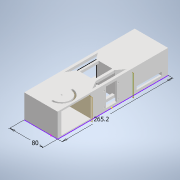
# Autodesk Inventor part: Part1
Saved by Autodesk Inventor 2022 (Build 260153000, 153)
## iProperties
Created: 2022-04-28
Part Number: Part1
Material: Generic
Document SubType Name: Modeling
Designer: Oana
Density: 1 g/cm^3
Appearance: Default
Author: Oana
Autodesk Inventor part; units mm, degrees
sketch "Sketch1" plane through (0, 0, 0) normal (0, 1, 0) x (-1, 0, 0)
  line L0 (49.8413, 129.2399) -> (-30.1587, 129.2399)
  line L1 (-30.1587, 129.2399) -> (-30.1587, -135.9601)
  line L2 (-30.1587, -135.9601) -> (49.8413, -135.9601)
  line L3 (49.8413, -135.9601) -> (49.8413, 129.2399)
  point P0 (0, 0)
  dimension "d0" = 265.2
  dimension "d1" = 80
  constraints: 8 end point, 2 parallel, 1 horizontal, 1 perpendicular
  measures "d0" distance of L0.end L1.end
  measures "d1" distance of L0.start L0.end
extrude "Extrusion1" add sketch "Sketch1" along normal blind 57
sketch "Sketch2" plane through (0, 0, 0) normal (0, -1, 0) x (1, 0, 0)
  line L0 (30.1587, 129.2399) -> (-49.8413, -135.9601) construction
  line L1 (30.1587, 129.2399) -> (30.1587, -135.9601) projected
  line L2 (-49.8413, 129.2399) -> (30.1587, 129.2399) projected
  line L3 (-49.8413, -135.9601) -> (-49.8413, 129.2399) projected
  line L4 (30.1587, -135.9601) -> (-49.8413, -135.9601) projected
  line L5 (-49.8413, 129.2399) -> (30.1587, -135.9601) construction
  line L6 (12.6587, 19.1399) -> (-32.3413, 19.1399)
  line L7 (-32.3413, 19.1399) -> (-32.3413, -25.8601)
  line L8 (-32.3413, -25.8601) -> (12.6587, -25.8601)
  line L9 (12.6587, -25.8601) -> (12.6587, 19.1399)
  line L10 (12.6587, 19.1399) -> (-32.3413, -25.8601) construction
  line L11 (-32.3413, 19.1399) -> (12.6587, -25.8601) construction
  point P0 (0, 0)
  point P1 (-9.8413, -3.3601)
  point P2 (-9.8413, -3.3601)
  dimension "d4" = 45
  dimension "d5" = 45
  constraints: 16 end point, 4 midpoint, 2 coincident, 2 parallel, 1 horizontal, 1 perpendicular
  measures "d4" distance of L6.start L6.end
  measures "d5" distance of L6.end L7.end
extrude "Extrusion2" cut sketch "Sketch2" against normal up to surface (57 mm away) contours L9 L8 L7 L6
sketch "Sketch6" plane through (0, 0, 0) normal (0, -1, 0) x (1, 0, 0)
  point P0 (0, 0)
sketch "Sketch7" plane through (0, 0, 0) normal (0, -1, 0) x (1, 0, 0)
  line L0 (12.4515, 19.3223) -> (12.4515, -25.5803)
  line L1 (12.4515, -25.5803) -> (30.1794, -49.7663)
  line L2 (30.1794, -49.7663) -> (30.1794, 50.0541)
  line L3 (30.1794, 50.0541) -> (12.4515, 19.3223)
  line L4 (-32.3413, 19.1399) -> (12.6587, 19.1399) projected
  line L5 (12.6587, 19.1399) -> (12.6587, -25.8601) projected
  line L6 (12.6587, -25.8601) -> (-32.3413, -25.8601) projected
  line L7 (-32.3413, -25.8601) -> (-32.3413, 19.1399) projected
  line L8 (30.1587, 129.2399) -> (30.1587, -135.9601) projected
  line L9 (-49.8413, 129.2399) -> (30.1587, 129.2399) projected
  line L10 (-49.8413, -135.9601) -> (-49.8413, 129.2399) projected
  line L11 (30.1587, -135.9601) -> (-49.8413, -135.9601) projected
  line L12 (-49.8413, 129.2399) -> (-49.8413, -135.9601)
  line L13 (-49.8413, -135.9601) -> (-49.8413, 129.2399) projected
  point P0 (0, 0)
  point P1 (12.6565, -25.8601)
  point P2 (30.1587, -49.7381)
  point P3 (30.1587, 50.0182)
  point P4 (12.4515, 19.1399)
  constraints: 10 end point, 1 collinear, 1 parallel, 1 vertical
extrude "Extrusion3" cut sketch "Sketch7" against normal up to surface (57 mm away) contours L3 L8 L1 L5 L4 L0
sketch "Sketch8" plane through (-32.3413, 0, 19.1399) normal (0, 0, -1) x (-1, 0, 0)
  line L0 (-44.7927, 0) -> (-38.7927, 0)
  line L1 (-38.7927, 0) -> (-38.7927, 6)
  line L2 (-38.7927, 6) -> (-44.7927, 6)
  line L3 (-44.7927, 6) -> (-44.7927, 0)
  line L4 (-44.7927, 51) -> (-38.7927, 51)
  line L5 (-38.7927, 51) -> (-38.7927, 57)
  line L6 (-38.7927, 57) -> (-44.7927, 57)
  line L7 (-44.7927, 57) -> (-44.7927, 51)
  line L8 (0, 0) -> (-44.7927, 0) projected
  point P0 (-32.3413, 0)
  dimension "d12" = 6
  dimension "d13" = 6
  constraints: 16 end point, 5 parallel, 2 equal length, 2 horizontal, 2 perpendicular, 2 point on line, 1 coincident
  measures "d12" distance of L0.end L1.end
  measures "d13" distance of L1.end L2.end
extrude "Extrusion4" add sketch "Sketch8" along normal up to surface (45 mm away)
sketch "Sketch9" plane through (-32.3413, 0, 19.1399) normal (1, 0, 0) x (0, 0, -1)
  line L0 (0, 57) -> (45, 57) projected
  line L1 (0, 0) -> (0, 57) projected
  line L2 (45, 0) -> (0, 0) projected
  line L3 (45, 0) -> (45, 57) projected
  line L4 (0, 0) -> (45, 0)
  line L5 (45, 0) -> (45, 57)
  line L6 (45, 57) -> (0, 57)
  line L7 (0, 57) -> (0, 0)
  point P0 (19.1399, 0)
  constraints: 8 end point, 2 parallel, 1 horizontal, 1 perpendicular
sketch "Sketch10" plane through (0, 0, 0) normal (0, -1, 0) x (1, 0, 0)
  line L0 (6.4515, -25.8601) -> (-32.3413, -25.8601) projected
  line L1 (-32.3413, -25.8601) -> (-32.3413, 19.1399) projected
  line L2 (-32.3413, 19.1399) -> (6.4515, 19.1399) projected
  line L3 (6.4515, 19.1399) -> (6.4515, -25.8601) projected
  line L4 (12.4515, -25.8601) -> (12.4515, 19.3223) projected
  line L5 (12.4515, 19.3223) -> (30.1587, 50.0182) projected
  line L6 (30.1587, 129.2399) -> (30.1587, 50.0182) projected
  line L7 (-49.8413, 129.2399) -> (30.1587, 129.2399) projected
  line L8 (-49.8413, -135.9601) -> (-49.8413, 129.2399) projected
  line L9 (30.1587, -135.9601) -> (-49.8413, -135.9601) projected
  line L10 (30.1587, -49.7381) -> (30.1587, -135.9601) projected
  line L11 (30.1587, -49.7381) -> (12.6565, -25.8601) projected
  line L12 (12.6565, -25.8601) -> (12.4515, -25.8601) projected
  line L13 (30.1587, 50.0182) -> (-49.8413, 50.0182) construction
  line L14 (30.1587, -49.7381) -> (-49.8413, -49.7381) construction
  line L15 (-32.3413, -25.8601) -> (-49.8413, -49.7381)
  line L16 (-49.8413, 50.0182) -> (-32.3413, 19.1399)
  line L17 (-49.8413, 50.0182) -> (-49.8413, -49.7381)
  point P0 (0, 0)
  constraints: 10 end point, 3 perpendicular, 2 point on line
extrude "Extrusion5" cut sketch "Sketch10" against normal up to surface (57 mm away) contours L15 L8 L16 L1
sketch "Sketch11" plane through (12.4515, 51, 19.1399) normal (0, 0, -1) x (-1, 0, 0)
  line L0 (44.7927, -51) -> (38.7927, -51)
  line L1 (38.7927, -51) -> (38.7927, -45)
  line L2 (38.7927, -45) -> (44.7927, -45)
  line L3 (44.7927, -45) -> (44.7927, -51)
  line L4 (44.7927, 6) -> (38.7927, 6)
  line L5 (38.7927, 6) -> (38.7927, 0)
  line L6 (38.7927, 0) -> (44.7927, 0)
  line L7 (44.7927, 0) -> (44.7927, 6)
  point P0 (12.4515, -51)
  dimension "d18" = 6
  dimension "d19" = 6
  dimension "d20" = 6
  dimension "d21" = 6
  constraints: 16 end point, 4 parallel, 2 horizontal, 2 perpendicular, 1 coincident
  measures "d18" distance of L0.end L1.end
  measures "d19" distance of L1.end L2.end
  measures "d20" distance of L4.end L5.end
  measures "d21" distance of L5.end L6.end
extrude "Extrusion6" add sketch "Sketch11" along normal up to surface (45 mm away)
ref_plane "Work Plane4" through (30.1587, 0, -49.7381) normal (0, 0, -1) x (0, -1, 0)
ref_plane "Work Plane5" through (30.1587, 0, 50.0182) normal (0, 0, 1) x (0, 1, 0)
sketch "Sketch14" plane through (30.1587, 0, -49.7381) normal (0, 0, -1) x (0, -1, 0)
  line L0 (-57, 17.5022) -> (-57, 0) projected
  line L1 (0, 17.5022) -> (-57, 17.5022) projected
  line L2 (0, 0) -> (0, 17.5022) projected
  line L3 (-57, 0) -> (0, 0) projected
  line L4 (-57, 0) -> (-51, 0)
  line L5 (-51, 0) -> (-51, 6)
  line L6 (-51, 6) -> (-57, 6)
  line L7 (-57, 6) -> (-57, 0)
  line L8 (-6, 0) -> (0, 0)
  line L9 (0, 0) -> (0, 6)
  line L10 (0, 6) -> (-6, 6)
  line L11 (-6, 6) -> (-6, 0)
  line L12 (0, 80) -> (-6, 80)
  line L13 (-6, 80) -> (-6, 74)
  line L14 (-6, 74) -> (0, 74)
  line L15 (0, 74) -> (0, 80)
  line L16 (-51, 80) -> (-57, 80)
  line L17 (-57, 80) -> (-57, 74)
  line L18 (-57, 74) -> (-51, 74)
  line L19 (-51, 74) -> (-51, 80)
  point P0 (0, 30.1587)
  dimension "d26" = 6
  dimension "d27" = 6
  dimension "d28" = 6
  dimension "d29" = 6
  constraints: 32 end point, 8 parallel, 8 perpendicular, 4 horizontal, 2 coincident
  measures "d26" distance of L4.end L5.end
  measures "d27" distance of L2.start L9.end
  measures "d28" distance of L12.end L13.end
  measures "d29" distance of L16.end L17.end
extrude "Extrusion7" add sketch "Sketch14" against normal up to surface (99.7563 mm away) contours L6 L5 L3 L0 | L2 L3 L11 L10 | L15 L14 L13 L12 | L19 L18 L17 L16
sketch "Sketch21" plane through (0, 0, 0) normal (0, -1, 0) x (1, 0, 0)
  arc A0 (-47.9413, -132.9601) -> (-44.9413, -135.9601) centre (-44.9413, -132.9601) ccw projected
  line L0 (-44.9413, -135.9601) -> (5.0587, -135.9601) projected
  arc A1 (5.0587, -135.9601) -> (8.0587, -132.9601) centre (5.0587, -132.9601) ccw projected
  line L1 (8.0587, -132.9601) -> (8.0587, -53.9601) projected
  arc A2 (8.0587, -53.9601) -> (5.0587, -50.9601) centre (5.0587, -53.9601) ccw projected
  line L2 (5.0587, -50.9601) -> (-44.9413, -50.9601) projected
  arc A3 (-44.9413, -50.9601) -> (-47.9413, -53.9601) centre (-44.9413, -53.9601) ccw projected
  line L3 (-47.9413, -53.9601) -> (-47.9413, -132.9601) projected
  spline S0 degree 3 poles (-15.1644, -62.5888) (-14.9628, -63.1953) (-14.6769, -64.3948) (-15.1993, -65.5952) (-15.7394, -65.8388) knots 0 0 0 0 0.539089 1 1 1 1 projected
  spline S1 degree 3 poles (-15.7394, -65.8388) (-14.4693, -66.5079) (-14.7995, -68.1116) (-15.2394, -69.1388) knots 0 0 0 0 1 1 1 1 projected
  spline S2 degree 3 poles (-15.2394, -69.1388) (-16.1604, -69.2836) (-17.1544, -68.892) (-17.7144, -68.1388) knots 0 0 0 0 1 1 1 1 projected
  spline S3 degree 3 poles (-17.7144, -68.1388) (-17.9663, -68.6471) (-18.6013, -68.8732) (-19.1394, -68.7888) knots 0 0 0 0 1 1 1 1 projected
  spline S4 degree 3 poles (-19.1394, -68.7888) (-19.3594, -69.0176) (-20.0467, -69.6983) (-21.1976, -69.5489) (-21.5644, -69.0067) knots 0 0 0 0 0.345385 1 1 1 1 projected
  spline S5 degree 3 poles (-21.5644, -69.0067) (-21.9665, -68.9706) (-23.0457, -68.9083) (-23.514, -67.8261) (-23.7411, -67.3609) knots 0 0 0 0 0.419509 1 1 1 1 projected
  spline S6 degree 3 poles (-23.7411, -67.3609) (-24.0812, -66.9137) (-24.6116, -66.2331) (-24.5516, -64.8465) (-23.8079, -64.3989) (-23.6675, -63.9025) knots 0 0 0 0 0.443124 0.609881 1 1 1 1 projected
  spline S7 degree 3 poles (-23.6675, -63.9025) (-23.3929, -62.9134) (-22.3359, -62.5853) (-21.4542, -62.4791) knots 0 0 0 0 1 1 1 1 projected
  spline S8 degree 3 poles (-21.4542, -62.4791) (-21.1982, -62.1521) (-20.2445, -61.9787) (-19.4136, -62.3867) (-19.1394, -62.8138) knots 0 0 0 0 0.450152 1 1 1 1 projected
  spline S9 degree 3 poles (-19.1394, -62.8138) (-18.555, -62.7473) (-17.9628, -63.0855) (-17.6144, -63.5388) knots 0 0 0 0 1 1 1 1 projected
  spline S10 degree 3 poles (-17.6144, -63.5388) (-17.3473, -63.1639) (-16.5978, -62.576) (-15.6276, -62.4003) (-15.1644, -62.5888) knots 0 0 0 0 0.487296 1 1 1 1 projected
  circle A4 centre (-2.8513, -113.7301) radius 0.8 projected
  circle A5 centre (-2.8513, -111.1901) radius 0.8 projected
  line L4 (0.4887, -111.9901) -> (-1.1113, -111.9901) projected
  line L5 (-1.1113, -111.9901) -> (-1.1113, -110.3901) projected
  line L6 (-1.1113, -110.3901) -> (0.4887, -110.3901) projected
  line L7 (0.4887, -110.3901) -> (0.4887, -111.9901) projected
  circle A6 centre (-0.3113, -113.7301) radius 0.8 projected
  line L8 (1.8687, -57.9101) -> (7.2487, -57.9101) projected
  line L9 (7.2487, -57.9101) -> (7.2487, -109.0101) projected
  line L10 (7.2487, -109.0101) -> (2.3859, -109.0101) projected
  line L11 (2.3859, -109.0101) -> (1.8687, -108.4929) projected
  line L12 (1.8687, -108.4929) -> (1.8687, -57.9101) projected
  circle A7 centre (-44.4413, -112.4601) radius 3 projected
  circle A8 centre (-44.4413, -54.4601) radius 3 projected
  circle A9 centre (4.5587, -54.4601) radius 3 projected
  circle A10 centre (4.5587, -112.4601) radius 3 projected
  line L13 (24.1587, -41.5524) -> (12.6565, -25.8601) projected
  line L14 (12.6565, -25.8601) -> (12.4515, -25.8601) projected
  line L15 (12.4515, -25.8601) -> (12.4515, 19.3223) projected
  line L16 (12.4515, 19.3223) -> (24.1587, 39.6171) projected
  line L17 (24.1587, -41.5524) -> (24.1587, 39.6171) projected
  line L18 (-43.8413, 39.4314) -> (-32.3413, 19.1399) projected
  line L19 (-32.3413, 19.1399) -> (-32.3413, -25.8601) projected
  line L20 (-32.3413, -25.8601) -> (-43.8413, -41.5513) projected
  line L21 (-43.8413, -41.5513) -> (-43.8413, 39.4314) projected
  line L22 (-26.3413, 19.1399) -> (-26.3413, -25.8601) projected
  line L23 (-26.3413, 19.1399) -> (6.4515, 19.1399) projected
  line L24 (6.4515, 19.1399) -> (6.4515, -25.8601) projected
  line L25 (6.4515, -25.8601) -> (-26.3413, -25.8601) projected
  line L26 (30.1587, 129.2399) -> (30.1587, -135.9601) projected
  line L27 (-49.8413, 129.2399) -> (30.1587, 129.2399) projected
  line L28 (-49.8413, -135.9601) -> (-49.8413, 129.2399) projected
  line L29 (30.1587, -135.9601) -> (-49.8413, -135.9601) projected
  line L30 (-49.8413, -45.9601) -> (20.1587, -45.9601)
  line L31 (20.1587, -45.9601) -> (20.1587, -135.9601)
  line L32 (20.1587, -135.9601) -> (-49.8413, -135.9601)
  line L33 (-49.8413, -135.9601) -> (-49.8413, -45.9601)
  point P0 (0, 0)
  dimension "d45" = 90
  dimension "d56" = 70
  constraints: 8 end point, 2 parallel, 2 point on line, 1 horizontal, 1 perpendicular
  measures "d45" distance of L30.end L31.end
  measures "d56" distance of L30.start L30.end
extrude "Extrusion12" cut sketch "Sketch21" against normal blind 25 contours L3 A3 L2 A2 L1 A1 L0 A0 | A0 L29 L28 L30 L31 A1 L1 A2 L2 A3 L3 | S0 S1 S2 S3 S4 S5 S6 S7 S8 S9 S10 | A4 | A5 | L4 L5 L6 L7 | A6 | L8 L9 L10 L11 L12 | A7 | A8 | A9 | A10
sketch "Sketch24" plane through (0, 0, 0) normal (0, -1, 0) x (1, 0, 0)
  line L0 (20.1587, -45.9601) -> (20.1587, -135.9601) projected
  line L1 (30.1587, -135.9601) -> (20.1587, -135.9601) projected
  line L2 (30.1587, 129.2399) -> (30.1587, -135.9601) projected
  line L3 (-49.8413, 129.2399) -> (30.1587, 129.2399) projected
  line L4 (-49.8413, -45.9601) -> (-49.8413, 129.2399) projected
  line L5 (-49.8413, -45.9601) -> (20.1587, -45.9601) projected
  line L6 (24.1587, -41.5524) -> (12.6565, -25.8601) projected
  line L7 (12.6565, -25.8601) -> (12.4515, -25.8601) projected
  line L8 (12.4515, -25.8601) -> (12.4515, 19.3223) projected
  line L9 (12.4515, 19.3223) -> (24.1587, 39.6171) projected
  line L10 (24.1587, -41.5524) -> (24.1587, 39.6171) projected
  line L11 (-43.8413, 39.4314) -> (-32.3413, 19.1399) projected
  line L12 (-32.3413, 19.1399) -> (-32.3413, -25.8601) projected
  line L13 (-32.3413, -25.8601) -> (-43.8413, -41.5513) projected
  line L14 (-43.8413, -41.5513) -> (-43.8413, 39.4314) projected
  line L15 (-26.3413, 19.1399) -> (-26.3413, -25.8601) projected
  line L16 (-26.3413, 19.1399) -> (6.4515, 19.1399) projected
  line L17 (6.4515, 19.1399) -> (6.4515, -25.8601) projected
  line L18 (6.4515, -25.8601) -> (-26.3413, -25.8601) projected
  line L19 (20.1587, -45.9601) -> (26.1587, -45.9601)
  line L20 (26.1587, -45.9601) -> (26.1587, -135.9601)
  line L21 (26.1587, -135.9601) -> (20.1587, -135.9601)
  line L22 (20.1587, -135.9601) -> (20.1587, -45.9601)
  point P0 (0, 0)
  dimension "d46" = 6
  constraints: 8 end point, 2 parallel, 1 horizontal, 1 perpendicular, 1 point on line
  measures "d46" distance between parallel lines of L20 L0
extrude "Extrusion13" cut sketch "Sketch24" against normal blind 7 contours L19 L20 L1 L0
ref_plane "Work Plane6" through (6.4515, 8.5, -23.3601) normal (1, 0, 0) x (0, 1, 0)
sketch "Sketch27" plane through (6.4515, 0, -25.8601) normal (-1, 0, 0) x (0, 0, 1)
  circle A0 centre (38.4706, 10.5294) radius 1 projected
  circle A1 centre (4.5294, 10.5294) radius 1 projected
  circle A2 centre (4.5294, 44.4706) radius 1 projected
  circle A3 centre (38.4706, 44.4706) radius 1 projected
  arc A4 (37.2331, 41.4654) -> (35.4654, 43.2331) centre (36.3492, 42.3492) ccw projected
  arc A5 (35.1118, 42.8796) -> (36.8796, 41.1118) centre (35.9957, 41.9957) ccw projected
  line L0 (37.2331, 41.4654) -> (36.8796, 41.1118) projected
  line L1 (35.1118, 42.8796) -> (35.4654, 43.2331) projected
  arc A6 (6.1204, 41.1118) -> (7.8882, 42.8796) centre (7.0043, 41.9957) ccw projected
  line L2 (6.1204, 41.1118) -> (5.7669, 41.4654) projected
  arc A7 (7.5346, 43.2331) -> (5.7669, 41.4654) centre (6.6508, 42.3492) ccw projected
  line L3 (7.5346, 43.2331) -> (7.8882, 42.8796) projected
  arc A8 (5.7669, 13.5346) -> (7.5346, 11.7669) centre (6.6508, 12.6508) ccw projected
  arc A9 (7.8882, 12.1204) -> (6.1204, 13.8882) centre (7.0043, 13.0043) ccw projected
  line L4 (5.7669, 13.5346) -> (6.1204, 13.8882) projected
  line L5 (7.8882, 12.1204) -> (7.5346, 11.7669) projected
  arc A10 (35.4654, 11.7669) -> (37.2331, 13.5346) centre (36.3492, 12.6508) ccw projected
  arc A11 (36.8796, 13.8882) -> (35.1118, 12.1204) centre (35.9957, 13.0043) ccw projected
  line L6 (35.4654, 11.7669) -> (35.1118, 12.1204) projected
  line L7 (36.8796, 13.8882) -> (37.2331, 13.5346) projected
  point P0 (25.8601, 0)
  constraints: 1 other
extrude "Extrusion16" cut sketch "Sketch27" against normal up to surface (6 mm away)
sketch "Sketch28" plane through (30.1587, 0, 129.2399) normal (1, 0, 0) x (0, 0, -1)
  point P0 (129.2399, 0)
sketch "Sketch29" plane through (0, 25, 0) normal (0, -1, 0) x (1, 0, 0)
  line L0 (-49.8413, -49.7381) -> (-47.0724, -45.9601) projected
  line L1 (-49.8413, -135.9601) -> (-49.8413, -49.7381) projected
  line L2 (20.1587, -135.9601) -> (-49.8413, -135.9601) projected
  line L3 (20.1587, -45.9601) -> (20.1587, -135.9601) projected
  line L4 (-47.0724, -45.9601) -> (20.1587, -45.9601) projected
  line L5 (-49.8413, -135.9601) -> (-44.8413, -135.9601)
  line L6 (-44.8413, -135.9601) -> (-44.8413, -115.9601)
  line L7 (-49.8413, -120.9601) -> (-49.8413, -135.9601)
  line L8 (-49.8413, -49.7381) -> (-44.8413, -49.7381) construction
  line L9 (-44.8413, -49.7381) -> (-44.8413, -54.7381)
  line L10 (-49.8413, -54.7381) -> (-49.8413, -49.7381)
  line L11 (-49.8413, -49.7381) -> (-47.0724, -45.9601)
  line L12 (-44.8413, -45.9601) -> (-44.8413, -49.7381)
  line L13 (-44.8413, -115.9601) -> (-49.8413, -115.9601)
  line L14 (-44.8413, -54.7381) -> (-49.8413, -54.7381)
  line L15 (-37.0388, -135.9601) -> (-37.0388, -115.9601)
  line L16 (-37.0388, -115.9601) -> (-44.8413, -115.9601)
  line L17 (-44.8413, -135.9601) -> (-37.0388, -135.9601)
  point P0 (0, 0)
  dimension "d57" = 20
  dimension "d164" = 5
  dimension "d165" = 5
  dimension "d168" = 20
  constraints: 26 end point, 4 parallel, 4 perpendicular, 4 point on line, 3 horizontal, 2 vertical, 1 collinear
  measures "d57" distance of L5.end L6.end
  measures "d164" distance of L6.end L13.end
  measures "d165" distance of L8.end L9.end
  measures "d168" distance of L15.start L15.end
ref_plane "Work Plane7" through (-49.8413, 0, -135.9601) normal (0, -1, 0) x (1, 0, 0)
ref_plane "Work Plane8" through (-49.8413, 3, -135.9601) normal (0, 1, 0) x (0, 0, 1)
ref_plane "Work Plane9" through (-49.8413, 3, -135.9601) normal (0, 1, 0) x (0, 0, 1)
extrude "Extrusion19" add sketch "Sketch29" along normal up to surface (22 mm away) contours L0 L4 L12 L9 L14 L1 | L13 L6 L2 L1 | L16 L15 L2 L6
sketch "Sketch34" plane through (0, 25, 0) normal (0, -1, 0) x (1, 0, 0)
  circle A0 centre (-32.3413, -111.4601) radius 1.35 projected
  circle A1 centre (-32.3413, -53.4601) radius 1.35 projected
  circle A2 centre (16.6587, -53.4601) radius 1.35 projected
  circle A3 centre (16.6587, -111.4601) radius 1.35 projected
  point P0 (0, 0)
extrude "Extrusion21" cut sketch "Sketch34" against normal blind 12
sketch "Sketch38" plane through (30.1587, 0, 129.2399) normal (1, 0, 0) x (0, 0, -1)
  line L0 (69.2217, 3) -> (19.2217, 3)
  line L1 (19.2217, 3) -> (19.2217, 53)
  line L2 (19.2217, 53) -> (69.2217, 53)
  line L3 (69.2217, 53) -> (69.2217, 3)
  line L4 (0, 57) -> (265.2, 57) projected
  line L5 (0, 0) -> (0, 57) projected
  line L6 (0, 0) -> (265.2, 0) projected
  line L7 (265.2, 0) -> (265.2, 57) projected
  line L8 (178.978, 51) -> (79.2217, 51) projected
  line L9 (178.978, 51) -> (178.978, 6) projected
  line L10 (178.978, 6) -> (79.2217, 6) projected
  line L11 (79.2217, 6) -> (79.2217, 51) projected
  line L12 (64.2734, 53) -> (64.2734, 57)
  line L13 (79.2217, 20.8757) -> (69.2217, 20.8757)
  point P0 (129.2399, 0)
  dimension "d75" = 50
  dimension "d76" = 4
  dimension "d77" = 3
  dimension "d78" = 10
  constraints: 12 end point, 4 perpendicular, 4 point on line, 2 parallel, 1 horizontal
  measures "d75" distance of L1.end L2.end
  measures "d76" distance of L12.start L12.end
  measures "d77" distance between parallel lines of L6 L0
  measures "d78" distance of L13.start L13.end
extrude "Extrusion23" cut sketch "Sketch38" against normal up to surface (80 mm away) contours L0 L1 L2 L3
sketch "Sketch42" plane through (30.1587, 0, 129.2399) normal (1, 0, 0) x (0, 0, -1)
  line L0 (19.2217, 3) -> (19.2217, 53) projected
  line L1 (19.2217, 53) -> (69.2217, 53) projected
  line L2 (69.2217, 53) -> (69.2217, 3) projected
  line L3 (69.2217, 3) -> (19.2217, 3) projected
  line L4 (0, 57) -> (265.2, 57) projected
  line L5 (0, 0) -> (0, 57) projected
  line L6 (0, 0) -> (265.2, 0) projected
  line L7 (265.2, 0) -> (265.2, 57) projected
  line L8 (178.978, 51) -> (79.2217, 51) projected
  line L9 (178.978, 51) -> (178.978, 6) projected
  line L10 (178.978, 6) -> (79.2217, 6) projected
  line L11 (79.2217, 6) -> (79.2217, 51) projected
  line L12 (178.978, 0) -> (142.103, 0)
  line L13 (142.103, 0) -> (142.103, 57)
  line L14 (142.103, 57) -> (178.978, 57)
  line L15 (178.978, 57) -> (178.978, 0)
  line L16 (178.978, 26.2177) -> (178.978, 57)
  line L17 (116.0967, 0) -> (79.2217, 0)
  line L18 (79.2217, 0) -> (79.2217, 57)
  line L19 (79.2217, 57) -> (116.0967, 57)
  line L20 (116.0967, 57) -> (116.0967, 0)
  line L21 (79.2217, 28.5) -> (79.2217, 57)
  point P0 (129.2399, 0)
  point P1 (178.978, 6)
  dimension "d87" = 36.875
  constraints: 20 end point, 9 point on line, 4 parallel, 4 perpendicular, 2 horizontal, 1 collinear, 1 midpoint
  measures "d87" distance of L12.start L12.end
extrude "Extrusion26" add sketch "Sketch42" against normal blind 3 contours L4 L20 L8 L18 | L8 L20 L10 L11 | L18 L10 L20 L6 | L4 L15 L8 L13 | L8 L9 L10 L13 | L13 L10 L15 L6
sketch "Sketch43" plane through (30.1587, 0, 129.2399) normal (1, 0, 0) x (0, 0, -1)
  line L0 (142.103, 9.5) -> (146.074, 9.5)
  line L1 (0, 0) -> (265.2, 0) projected
  line L2 (142.103, 6) -> (142.103, 9.5)
  circle A0 centre (146.074, 9.5) radius 1.5
  point P0 (129.2399, 0)
  dimension "d90" = 3.971
  dimension "d91" = 3.5
  dimension "d92" = 3
  constraints: 4 end point, 2 coincident, 1 centre point, 1 horizontal, 1 parallel, 1 vertical
  measures "d90" distance of L0.start L0.end
  measures "d91" distance of L2.start L0.start
  measures "d92" diameter of A0
extrude "Extrusion27" cut sketch "Sketch43" against normal up to surface (3 mm away)
sketch "Sketch44" plane through (27.1587, 0, 129.2399) normal (-1, 0, 0) x (0, 0, 1)
  circle A0 centre (-112.1329, 9.5) radius 1 projected
  circle A1 centre (-112.1329, 43.4411) radius 1 projected
  point P0 (-129.2399, 0)
extrude "Extrusion28" cut sketch "Sketch44" against normal up to surface (3 mm away)
sketch "Sketch45" plane through (27.1587, 0, 129.2399) normal (-1, 0, 0) x (0, 0, 1)
  circle A0 centre (-146.074, 43.4411) radius 1 projected
  point P0 (-129.2399, 0)
extrude "Extrusion29" cut sketch "Sketch45" against normal up to surface (3 mm away)
sketch "Sketch54" plane through (30.1587, 0, 129.2399) normal (1, 0, 0) x (0, 0, -1)
  line L0 (249.9086, 6.9208) -> (189.9086, 6.9208)
  line L1 (189.9086, 6.9208) -> (189.9086, 14.9208)
  line L2 (189.9086, 14.9208) -> (249.9086, 14.9208)
  line L3 (249.9086, 14.9208) -> (249.9086, 6.9208)
  point P0 (129.2399, 0)
  dimension "d128" = 8
  dimension "d131" = 60
  constraints: 8 end point, 2 parallel, 1 horizontal, 1 perpendicular
  measures "d128" distance between parallel lines of L2 L0
  measures "d131" distance of L1.end L2.end
extrude "Extrusion37" cut sketch "Sketch54" against normal blind 10
sketch "Sketch55" plane through (30.1587, 0, 129.2399) normal (1, 0, 0) x (0, 0, -1)
  circle A0 centre (112.1329, 43.4411) radius 1 projected
  circle A1 centre (112.1329, 9.5) radius 1 projected
  circle A2 centre (146.074, 9.5) radius 1.5 projected
  circle A3 centre (146.074, 43.4411) radius 1 projected
  circle A4 centre (112.1329, 43.4411) radius 1.5
  circle A5 centre (112.1329, 9.5) radius 1.5
  circle A6 centre (146.074, 9.5) radius 1.5
  circle A7 centre (146.074, 43.4411) radius 1.5
  point P0 (129.2399, 0)
  dimension "d132" = 3
  dimension "d133" = 3
  dimension "d134" = 3
  dimension "d135" = 3
  constraints: 4 centre point, 4 coincident
  measures "d132" diameter of A4
  measures "d133" diameter of A5
  measures "d134" diameter of A6
  measures "d135" diameter of A7
extrude "Extrusion38" cut sketch "Sketch55" against normal up to surface (3 mm away) contours A0 | A1 | A2 | A3 | A4 | A5 | A7
sketch "Sketch56" plane through (30.1587, 0, 129.2399) normal (1, 0, 0) x (0, 0, -1)
  point P0 (129.2399, 0)
sketch "Sketch58" plane through (0, 0, 0) normal (0, -1, 0) x (1, 0, 0)
  line L0 (-15.7732, 129.2399) -> (-15.7732, 49.7366)
  line L1 (-49.8413, 129.2399) -> (30.1587, 129.2399) projected
  point P0 (0, 0)
  point P1 (15.1587, 129.2399)
  constraints: 2 end point, 1 point on line, 1 vertical
sketch "Sketch61" plane through (0, 57, 0) normal (0, 1, 0) x (1, 0, 0)
  line L0 (-43.8413, 41.5513) -> (-43.8413, -39.4314) projected
  line L1 (-43.8413, 41.5513) -> (-32.3413, 25.8601) projected
  line L2 (-32.3413, -19.1399) -> (-32.3413, 25.8601) projected
  line L3 (-32.3413, -19.1399) -> (-43.8413, -39.4314) projected
  line L4 (-26.3413, 25.8601) -> (6.4515, 25.8601) projected
  line L5 (6.4515, -19.1399) -> (6.4515, 25.8601) projected
  line L6 (6.4515, -19.1399) -> (-26.3413, -19.1399) projected
  line L7 (-26.3413, -19.1399) -> (-26.3413, 25.8601) projected
  line L8 (30.1587, -129.2399) -> (30.1587, 135.9601) projected
  line L9 (30.1587, 135.9601) -> (-49.8413, 135.9601) projected
  line L10 (-49.8413, 135.9601) -> (-49.8413, -129.2399) projected
  line L11 (-49.8413, -129.2399) -> (30.1587, -129.2399) projected
  line L12 (24.1587, -39.6171) -> (12.4515, -19.3223) projected
  line L13 (12.4515, -19.3223) -> (12.4515, 25.8601) projected
  line L14 (12.4515, 25.8601) -> (12.6565, 25.8601) projected
  line L15 (12.6565, 25.8601) -> (24.1587, 41.5524) projected
  line L16 (24.1587, 41.5524) -> (24.1587, -39.6171) projected
  line L17 (0.1587, -50.0182) -> (0.1587, -68.0309)
  line L18 (46.1587, -50.0182) -> (-65.8413, -50.0182) projected
  arc A0 (0.1587, -64.0309) -> (0.1587, -115.0309) centre (0.1587, -89.5309) ccw construction
  arc A1 (0.1587, -115.0309) -> (0.1587, -64.0309) centre (0.1587, -89.5309) ccw
  line L19 (0.1587, -115.0309) -> (0.1587, -129.2399)
  arc A2 (0.1587, -111.0309) -> (0.1587, -68.0309) centre (0.1587, -89.5309) ccw
  line L20 (0.1587, -68.0309) -> (0.1587, -115.0309)
  arc A3 (0.1587, -68.0309) -> (0.1587, -111.0309) centre (0.1587, -89.5309) ccw construction
  line L21 (0.1587, -68.0309) -> (0.1587, -64.0309)
  line L22 (0.1587, -115.0309) -> (0.1587, -111.0309)
  circle A4 centre (0.1587, -89.5309) radius 1.5
  point P0 (0, 0)
  dimension "d148" = 30
  dimension "d149" = 51
  dimension "d150" = 43
  dimension "d153" = 3
  dimension "d154" = 25.5
  constraints: 10 end point, 10 point on circle, 5 centre point, 4 point on line, 3 coincident, 3 perpendicular, 2 vertical
  measures "d148" distance between parallel lines of L17 L8
  measures "d149" distance of L19.start L21.end
  measures "d150" diameter of A2
  measures "d153" diameter of A4
  measures "d154" distance of A2.centre L21.end
extrude "Extrusion41" cut sketch "Sketch61" against normal up to surface (4 mm away) contours L20 A2 L17 A1 | A4 L20 | L20 A4
sketch "Sketch62" plane through (30.1587, 0, 129.2399) normal (1, 0, 0) x (0, 0, -1)
  circle A0 centre (112.1329, 43.4411) radius 1.5 projected
  circle A1 centre (146.074, 43.4411) radius 1.5 projected
  circle A2 centre (112.1329, 9.5) radius 1.5 projected
  line L0 (189.9086, 6.9208) -> (189.9086, 14.9208) projected
  line L1 (189.9086, 14.9208) -> (249.9086, 14.9208) projected
  line L2 (249.9086, 14.9208) -> (249.9086, 6.9208) projected
  line L3 (249.9086, 6.9208) -> (189.9086, 6.9208) projected
  circle A3 centre (146.074, 9.5) radius 1.5 projected
  line L4 (0, 0) -> (265.2, 0) projected
  line L5 (265.2, 0) -> (265.2, 57) projected
  line L6 (0, 57) -> (265.2, 57) projected
  line L7 (0, 0) -> (0, 57) projected
  line L8 (19.2217, 3) -> (19.2217, 53) projected
  line L9 (19.2217, 53) -> (69.2217, 53) projected
  line L10 (69.2217, 53) -> (69.2217, 3) projected
  line L11 (69.2217, 3) -> (19.2217, 3) projected
  line L12 (116.0967, 6) -> (116.0967, 51) projected
  line L13 (142.103, 51) -> (116.0967, 51) projected
  line L14 (142.103, 51) -> (142.103, 6) projected
  line L15 (142.103, 6) -> (116.0967, 6) projected
  line L16 (19.2217, 53) -> (9.2217, 53)
  line L17 (9.2217, 53) -> (9.2217, 3)
  line L18 (9.2217, 3) -> (19.2217, 3)
  line L19 (19.2217, 3) -> (19.2217, 53)
  point P0 (129.2399, 0)
  dimension "d155" = 10
  constraints: 8 end point, 2 parallel, 1 horizontal, 1 perpendicular
  measures "d155" distance of L17.end L18.end
extrude "Extrusion42" cut sketch "Sketch62" against normal up to surface (80 mm away) contours L18 L17 L16 L8
sketch "Sketch63" plane through (30.1587, 0, 50.0182) normal (0, 0, 1) x (0, 1, 0)
  point P0 (0, 30.1587)
sketch "Sketch64" plane through (30.1587, 0, 129.2399) normal (1, 0, 0) x (0, 0, -1)
  line L0 (116.0967, 6) -> (116.0967, 51) projected
  line L1 (142.103, 51) -> (116.0967, 51) projected
  line L2 (142.103, 51) -> (142.103, 6) projected
  line L3 (142.103, 6) -> (116.0967, 6) projected
  line L4 (69.2217, 3) -> (9.2217, 3) projected
  line L5 (9.2217, 3) -> (9.2217, 53) projected
  line L6 (9.2217, 53) -> (69.2217, 53) projected
  line L7 (69.2217, 53) -> (69.2217, 3) projected
  line L8 (0, 0) -> (265.2, 0) projected
  line L9 (265.2, 0) -> (265.2, 57) projected
  line L10 (0, 57) -> (265.2, 57) projected
  line L11 (0, 0) -> (0, 57) projected
  circle A0 centre (146.074, 9.5) radius 1.5 projected
  line L12 (189.9086, 6.9208) -> (189.9086, 14.9208) projected
  line L13 (189.9086, 14.9208) -> (249.9086, 14.9208) projected
  line L14 (249.9086, 14.9208) -> (249.9086, 6.9208) projected
  line L15 (249.9086, 6.9208) -> (189.9086, 6.9208) projected
  circle A1 centre (112.1329, 9.5) radius 1.5 projected
  circle A2 centre (146.074, 43.4411) radius 1.5 projected
  circle A3 centre (112.1329, 43.4411) radius 1.5 projected
  line L16 (69.2217, 53) -> (79.3445, 53)
  line L17 (79.3445, 53) -> (79.3445, 3)
  line L18 (79.3445, 3) -> (69.2217, 3)
  line L19 (69.2217, 3) -> (69.2217, 53)
  point P0 (129.2399, 0)
  constraints: 8 end point, 2 parallel, 1 horizontal, 1 perpendicular
extrude "Extrusion43" cut sketch "Sketch64" against normal up to surface (80 mm away) contours L7 L16 L17 L18
sketch "Sketch65" plane through (-49.8413, 0, 129.2399) normal (-1, 0, 0) x (0, 0, 1)
  circle A0 centre (-252.7, 22.2932) radius 2.5
  line L0 (-265.2, 57) -> (0, 57) projected
  line L1 (-265.2, 0) -> (0, 0) projected
  line L2 (-265.2, 3) -> (-265.2, 57) projected
  line L3 (-252.7, 22.2932) -> (-265.2, 22.2932)
  line L4 (-265.2, 22.2932) -> (-265.2, 28.2932)
  line L5 (-265.2, 28.2932) -> (-265.2, 28.2932)
  line L6 (-265.2, 28.2932) -> (-265.2, 34.2932)
  line L7 (-265.2, 34.2932) -> (-252.7, 34.2932)
  circle A1 centre (-252.7, 34.2932) radius 2.5
  point P0 (-129.2399, 0)
  dimension "d161" = 5
  dimension "d181" = 12.5
  dimension "d182" = 6
  dimension "d183" = 6
  dimension "d184" = 5
  constraints: 10 end point, 4 perpendicular, 4 point on line, 2 centre point, 1 coincident, 1 horizontal, 1 parallel, 1 vertical, 1 other
  measures "d161" diameter of A0
  measures "d181" distance of L3.start L3.end
  measures "d182" distance of L4.start L4.end
  measures "d183" distance of L4.end L6.end
  measures "d184" diameter of A1
extrude "Extrusion44" cut sketch "Sketch65" against normal blind 12
sketch "Sketch66" plane through (-49.8413, 0, 129.2399) normal (-1, 0, 0) x (0, 0, 1)
  circle A0 centre (-252.7, 22.2932) radius 2.5 projected
  line L0 (-79.3445, 3) -> (-79.3445, 6) projected
  line L1 (-175.2, 6) -> (-79.3445, 6) projected
  line L2 (-175.2, 6) -> (-175.2, 0) projected
  line L3 (-175.2, 0) -> (0, 0) projected
  line L4 (0, 0) -> (0, 57) projected
  line L5 (-265.2, 57) -> (0, 57) projected
  line L6 (-265.2, 3) -> (-265.2, 57) projected
  line L7 (-245.2, 3) -> (-265.2, 3) projected
  line L8 (-245.2, 25) -> (-245.2, 3) projected
  line L9 (-245.2, 25) -> (-183.978, 25) projected
  line L10 (-183.978, 25) -> (-183.978, 3) projected
  line L11 (-178.978, 3) -> (-183.978, 3) projected
  line L12 (-178.978, 3) -> (-178.978, 51) projected
  line L13 (-178.978, 51) -> (-79.3445, 51) projected
  line L14 (-79.3445, 51) -> (-79.3445, 53) projected
  line L15 (-79.3445, 53) -> (-9.2217, 53) projected
  line L16 (-9.2217, 53) -> (-9.2217, 3) projected
  line L17 (-9.2217, 3) -> (-79.3445, 3) projected
  line L18 (-9.2217, 29.5326) -> (-17.2217, 29.5326) construction
  line L19 (-17.2217, 29.5326) -> (-17.2217, 13.5326)
  line L20 (-17.2217, 13.5326) -> (-9.2217, 13.5326)
  line L21 (-9.2217, 13.5326) -> (-9.2217, 29.5326)
  line L22 (-9.2217, 29.5326) -> (-17.2217, 29.5326)
  line L23 (-17.2217, 29.5326) -> (-17.2217, 45.5326)
  line L24 (-17.2217, 45.5326) -> (-9.2217, 45.5326)
  line L25 (-9.2217, 45.5326) -> (-9.2217, 29.5326)
  point P0 (-129.2399, 0)
  point P1 (-9.2217, 13.5326)
  point P2 (-9.2217, 45.5326)
  dimension "d169" = 8
  dimension "d170" = 16
  constraints: 16 end point, 4 parallel, 2 horizontal, 2 perpendicular, 2 point on line, 1 collinear
  measures "d169" distance of L19.end L20.end
  measures "d170" distance of L18.end L19.end
extrude "Extrusion45" add sketch "Sketch66" against normal blind 30 contours L20 L19 L22 L16 | L22 L23 L24 L16
sketch "Sketch67" plane through (-49.8413, 0, 129.2399) normal (-1, 0, 0) x (0, 0, 1)
  circle A0 centre (-252.7, 22.2932) radius 2.5 projected
  line L0 (-79.3445, 3) -> (-79.3445, 6) projected
  line L1 (-175.2, 6) -> (-79.3445, 6) projected
  line L2 (-175.2, 6) -> (-175.2, 0) projected
  line L3 (-175.2, 0) -> (0, 0) projected
  line L4 (0, 0) -> (0, 57) projected
  line L5 (-265.2, 57) -> (0, 57) projected
  line L6 (-265.2, 3) -> (-265.2, 57) projected
  line L7 (-245.2, 3) -> (-265.2, 3) projected
  line L8 (-245.2, 25) -> (-245.2, 3) projected
  line L9 (-245.2, 25) -> (-183.978, 25) projected
  line L10 (-183.978, 25) -> (-183.978, 3) projected
  line L11 (-178.978, 3) -> (-183.978, 3) projected
  line L12 (-178.978, 3) -> (-178.978, 51) projected
  line L13 (-178.978, 51) -> (-79.3445, 51) projected
  line L14 (-79.3445, 51) -> (-79.3445, 53) projected
  line L15 (-79.3445, 53) -> (-9.2217, 53) projected
  line L16 (-9.2217, 53) -> (-9.2217, 45.5326) projected
  line L17 (-9.2217, 45.5326) -> (-17.2217, 45.5326) projected
  line L18 (-17.2217, 45.5326) -> (-17.2217, 13.5326) projected
  line L19 (-17.2217, 13.5326) -> (-9.2217, 13.5326) projected
  line L20 (-9.2217, 13.5326) -> (-9.2217, 3) projected
  line L21 (-9.2217, 3) -> (-79.3445, 3) projected
  line L22 (0, 30) -> (-12.5, 30)
  line L23 (-12.5, 30) -> (-12.5, 36)
  line L24 (-12.5, 36) -> (-12.5, 30)
  line L25 (-12.5, 30) -> (-12.5, 24)
  circle A1 centre (-12.5, 24) radius 2.5
  circle A2 centre (-12.5, 36) radius 2.5
  point P0 (-129.2399, 0)
  point P1 (-17.2217, 30)
  dimension "d173" = 12.5
  dimension "d175" = 6
  dimension "d176" = 6
  dimension "d177" = 5
  dimension "d178" = 5
  constraints: 8 end point, 3 point on line, 2 centre point, 2 coincident, 1 collinear, 1 horizontal, 1 vertical
  measures "d173" distance of L22.start L22.end
  measures "d175" distance of L22.end L23.end
  measures "d176" distance of L22.end L25.end
  measures "d177" diameter of A1
  measures "d178" diameter of A2
extrude "Extrusion46" cut sketch "Sketch67" against normal blind 12 contours A1 | A2
sketch "Sketch68" plane through (30.1587, 3, 120.0182) normal (0, 0, -1) x (-1, 0, 0)
  point P0 (30.1587, -3)
body "Solid1"
